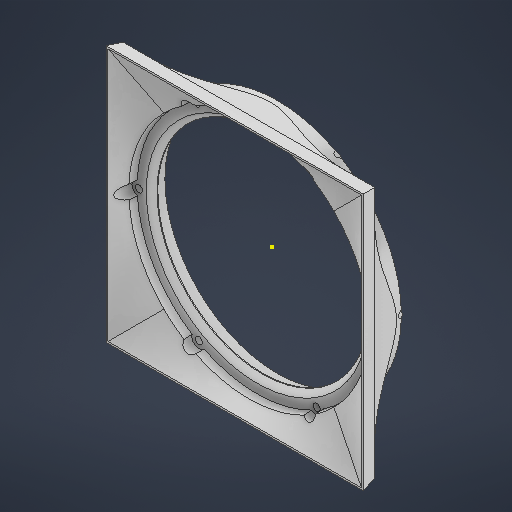
# Autodesk Inventor part: 供弹斜板
Saved by Autodesk Inventor 2025 (Build 290162000, 162)
## iProperties
Created: 2024-05-11
Part Number: 供弹斜板
Material: 常规
Document SubType Name: Modeling
Designer: HZD
Density: 1 g/cm^3
Appearance: 默认
Author: HZD
## iProperties of the stored document 供弹斜板_3D 打印.ipt
Created: 2024-07-10
Part Number: 供弹斜板_3D 打印
Material: 常规
Document SubType Name: Modeling
Designer: HZD
Density: 1 g/cm^3
Appearance: 默认
Author: HZD
Autodesk Inventor part; units mm, degrees
ref_plane "YZ Plane" through (0, 0, 0) normal (1, 0, 0) x (0, 1, 0)
ref_plane "XZ Plane" through (0, 0, 0) normal (0, 1, 0) x (-1, 0, 0)
ref_plane "工作平面1" through (0, 0, 20) normal (0, 0, 1) x (1, 0, 0)
sketch "草图30" plane through (-71.5017, -42.1486, 0) normal (0, 0, -1) x (-0.8614667, -0.5078141, 0)
  circle A0 centre (-83, 0) radius 64
  point P0 (-83, 0)
  dimension "d82" = 128
  constraints: 1 centre point, 1 coincident
  measures "d82" diameter of A0
sketch "草图19" plane through (0, 0, 3) normal (0, 0, 1) x (0.8718892, -0.4897032, 0)
  circle A0 centre (0, 0) radius 70.8 projected
  line L0 (-27.0916, -96.6485) -> (-93.2274, 21.1025)
  line L1 (98.0112, -26.2677) -> (-27.0916, -96.6485)
  line L2 (45.3823, -54.5376) -> (42.0698, -86.8145)
  line L3 (42.0698, -86.8145) -> (-27.0916, -96.6485)
  line L4 (-27.3263, -97.3539) -> (-18.3217, -65.2736) projected
  line L5 (-97.3643, 28.5723) -> (-27.1597, -96.6294)
  line L6 (-67.1338, -22.9554) -> (-81.1015, -52.2415)
  line L7 (-81.1015, -52.2415) -> (-27.1597, -96.6294)
  point P0 (34.788, -61.8361)
  point P1 (-61.8605, -34.7444)
  constraints: 14 end point, 4 symmetric about line, 4 other
sketch "草图21" plane through (-72.5, 72.5, 24) normal (0, 0, 1) x (1, 0, 0)
  circle A0 centre (72.5, -72.5) radius 70.95
  arc A1 (72.5499, -143.45) -> (1.55, -72.5) centre (72.5, -72.5) ccw projected
  line L0 (89.6905, -141.336) -> (42.9672, -149.9362)
  line L1 (42.9672, -149.9362) -> (-4.9362, -149.9362)
  line L2 (22.3308, -122.6692) -> (24.5608, -120.4392) projected
  line L3 (-4.9362, -149.9362) -> (22.3308, -122.6692)
  line L4 (3.664, -55.3095) -> (-4.9362, -102.0328)
  line L5 (-4.9362, -102.0328) -> (-4.9362, -149.9362)
  point P0 (80.9465, -142.9454)
  point P1 (2.0546, -64.0535)
  constraints: 10 end point, 2 symmetric about line, 1 centre point, 1 coincident, 1 horizontal, 1 point on circle
sketch "草图7" plane through (0, 0, 3) normal (0, 0, 1) x (1, 0, 0)
  circle A0 centre (-80.5933, -13.2719) radius 14.5326
  circle A1 centre (0, 0) radius 67.1463 projected
  constraints: 1 centre point, 1 tangent
sketch "草图2" plane through (0, 0, 0) normal (0, 0, 1) x (1, 0, 0)
  circle A0 centre (0, 0) radius 70
  dimension "d8" = 140
  constraints: 1 centre point, 1 coincident
  measures "d8" diameter of A0
sketch "草图3" plane through (0, 0, 20) normal (0, 0, 1) x (1, 0, 0)
  circle A0 centre (0, 0) radius 71
  dimension "d7" = 142
  constraints: 1 centre point, 1 coincident
  measures "d7" diameter of A0
loft "放样1" add profiles "草图2", "草图3"
shell "抽壳1" thickness 3 removed faces 1 at (12.047, 0, 20)
sketch "草图6" plane through (0, 0, 3) normal (0, 0, 1) x (1, 0, 0)
  circle A0 centre (0, 0) radius 63.4
  point P0 (0, 0)
  dimension "d97" = 126.8
  constraints: 1 centre point
  measures "d97" diameter of A0
extrude "拉伸2" cut sketch "草图6" against normal blind 38
sketch "草图9" plane through (0, 0, 20) normal (0, 0, 1) x (1, 0, 0)
  line L0 (71, 71) -> (-71, 71)
  line L1 (-71, 71) -> (-71, -71)
  line L2 (-71, -71) -> (71, -71)
  line L3 (71, -71) -> (71, 71)
  line L4 (71, 71) -> (-71, -71) construction
  line L5 (-71, 71) -> (71, -71) construction
  circle A0 centre (0, 0) radius 67.9963 projected
  dimension "d27" = 142
  dimension "d28" = 142
  constraints: 12 end point, 2 midpoint, 2 parallel, 1 horizontal, 1 perpendicular
  measures "d27" distance of L2.end L0.start
  measures "d28" distance of L0.start L0.end
extrude "拉伸4" add sketch "草图9" along normal blind 1
extrude "拉伸5" add sketch "草图9" against normal blind 4
fillet "圆角9" radius 19 1 edges at (-70.8, 0, 16)
ref_plane "工作平面2" through (0, 0, 24) normal (0, 0, 1) x (1, 0, 0)
sketch "草图12" plane through (0, 0, 16) normal (0, 0, -1) x (-1, 0, 0)
  line L0 (71, -71) -> (-71, -71) projected
  line L1 (71, 71) -> (-71, 71)
  line L2 (-71, 71) -> (-71, -71)
  line L3 (-71, -71) -> (71, -71)
  line L4 (71, -71) -> (71, 71)
  line L5 (71, 71) -> (-71, -71) construction
  line L6 (-71, 71) -> (71, -71) construction
  point P0 (0, 0)
  constraints: 12 end point, 2 midpoint, 2 parallel, 1 horizontal, 1 perpendicular
sketch "草图10" plane through (0, 0, 24) normal (0, 0, 1) x (1, 0, 0)
  line L0 (72.5, 72.5) -> (-72.5, 72.5)
  line L1 (-72.5, 72.5) -> (-72.5, -72.5)
  line L2 (-72.5, -72.5) -> (72.5, -72.5)
  line L3 (72.5, -72.5) -> (72.5, 72.5)
  line L4 (72.5, 72.5) -> (-72.5, -72.5) construction
  line L5 (-72.5, 72.5) -> (72.5, -72.5) construction
  point P0 (0, 0)
  dimension "d30" = 145
  dimension "d31" = 145
  constraints: 12 end point, 2 midpoint, 2 parallel, 1 horizontal, 1 perpendicular
  measures "d30" distance of L2.end L1.end
  measures "d31" distance of L0.end L1.end
loft "放样2" add profiles "草图12", "草图10"
sketch "草图13" plane through (-72.5, 72.5, 24) normal (0, 0, 1) x (1, 0, 0)
  line L0 (1, -1) -> (144, -1)
  line L1 (144, -1) -> (144, -144)
  line L2 (144, -144) -> (1, -144)
  line L3 (1, -144) -> (1, -1)
  line L4 (144, -1) -> (1, -1)
  line L5 (1, -1) -> (1, -144)
  line L6 (1, -144) -> (144, -144)
  line L7 (144, -144) -> (144, -1)
  line L8 (0, 0) -> (145, 0) projected
  line L9 (0, -145) -> (0, 0) projected
  line L10 (145, 0) -> (145, -145) projected
  line L11 (145, -145) -> (0, -145) projected
  point P0 (72.5, -72.5)
  dimension "d88" = 1
  dimension "d89" = 1
  dimension "d90" = 1
  dimension "d91" = 1
  constraints: 16 end point, 2 parallel, 1 horizontal, 1 perpendicular
  measures "d88" distance between parallel lines of L8 L0
  measures "d89" distance between parallel lines of L9 L3
  measures "d90" distance between parallel lines of L10 L1
  measures "d91" distance between parallel lines of L2 L11
sketch "草图15" plane through (0, 0, 16) normal (0, 0, -1) x (-1, 0, 0)
  circle A0 centre (0, 0) radius 67.7963 projected
  point P0 (0, 0)
loft "放样3" cut profiles "草图13", "草图15" contours L0 L1 L2 L3 / all
sketch "草图17" plane through (0, 0, 3) normal (0, 0, 1) x (1, 0, 0)
  circle A0 centre (33.7696, -57.2875) radius 2
  circle A1 centre (-32.7276, -57.8891) radius 2
  circle A2 centre (-66.4973, -0.6016) radius 2
  circle A3 centre (32.7276, 57.8891) radius 2
  circle A4 centre (66.4973, 0.6016) radius 1.65
  circle A5 centre (-33.7696, 57.2875) radius 1.65
  point P0 (0, 0)
  constraints: 6 centre point, 12 other
extrude "拉伸6" cut sketch "草图17" along normal mid plane 104
sketch "草图18" plane through (0, 0, 3) normal (0, 0, 1) x (0.8718892, -0.4897032, 0)
  point P0 (0, 0)
sketch "草图24" plane through (0, 0, 3) normal (0, 0, 1) x (0.8718892, -0.4897032, 0)
  circle A0 centre (0.1864, 66.4997) radius 2 projected
  circle A1 centre (0.1864, 66.4997) radius 4
  point P0 (0, 0)
  dimension "d63" = 8
  constraints: 1 centre point, 1 coincident
  measures "d63" diameter of A1
extrude "拉伸11" cut sketch "草图24" along normal blind 33.5 contours A0 | A1
pattern_circular "环形阵列1" count 6 over 360 about axis through (0, 0, -10) along (0, 0, 1) of "拉伸11"
sketch "草图27" plane through (0, 0, 3) normal (0, 0, 1) x (0.8614667, 0.5078141, 0)
  arc A0 (-58.8355, 37.0514) -> (-61.5194, 32.4983) centre (-57.5907, 33.25) ccw projected
  circle A1 centre (-57.5907, 33.25) radius 4
  circle A2 centre (0, 66.5) radius 1.65 projected
  circle A3 centre (0, 66.5) radius 4
  circle A4 centre (0, 0) radius 63.4 projected
  circle A5 centre (57.5907, 33.25) radius 2 projected
  circle A6 centre (57.5907, 33.25) radius 4.0042
  circle A7 centre (57.5907, -33.25) radius 1.65 projected
  circle A8 centre (57.5907, -33.25) radius 4
  circle A9 centre (0, -66.5) radius 2 projected
  circle A10 centre (0, -66.5) radius 4
  circle A11 centre (0, 0) radius 68.1203
  circle A12 centre (-57.5907, 33.25) radius 2 projected
  circle A13 centre (-57.5907, -33.25) radius 2 projected
  circle A14 centre (-57.5907, -33.25) radius 4.0197
  point P0 (0, 0)
  point P1 (60.759, 30.8014)
  point P2 (57.0543, 37.2181)
  point P3 (3.7, 68.0198)
  point P4 (-3.7, 68.0198)
  point P5 (-57.0568, 37.2142)
  point P6 (-58.8355, 37.0514)
  point P7 (-61.5194, 32.4983)
  point P8 (-60.7569, 30.8056)
  point P9 (-60.7667, -30.7862)
  point P10 (-57.0449, -37.2324)
  point P11 (-3.7, -68.0198)
  point P12 (3.7, -68.0198)
  point P13 (57.0568, -37.2142)
  point P14 (60.7569, -30.8056)
  point P15 (58.8357, -34.3328)
  point P16 (59.1509, -33.7868)
  point P17 (2.4678, 63.352)
  point P18 (56.0983, -29.5388)
  point P19 (53.6305, -33.8131)
  point P20 (-56.0983, 29.5388)
  point P21 (-53.6305, 33.8131)
  point P22 (-2.4678, 63.352)
  point P23 (-59.5783, 33.0274)
  point P24 (-58.3917, 35.0826)
  point P25 (-58.3917, -35.0826)
  point P26 (-59.5783, -33.0274)
  point P27 (-1.1866, -68.11)
  point P28 (1.1866, -68.11)
  point P29 (-0.3153, 68.1196)
  point P30 (0.3153, 68.1196)
  point P31 (58.3917, 35.0826)
  point P32 (59.5783, 33.0274)
  constraints: 7 coincident, 6 centre point, 2 horizontal alignment, 1 concentric, 4 other
extrude "拉伸15" add sketch "草图27" along normal blind 8.5 contours A1 A11 A12 A0 | A11 A3 A4 A1 | A1 A4 A11 A12 | A1 A4 A14 A11 | A11 A2 A3 A4 | A3 A11 A2 | A14 A4 A11 A13 | A11 A13 A14 | A11 A6 A4 A3 | A14 A4 A10 A11 | A11 A5 A6 A4 | A6 A11 A5 | A11 A9 A10 | A10 A4 A11 A9 | A10 A4 A8 A11 | A6 A11 A8 A4 | A11 A7 A8 | A8 A4 A11 A7
extrude "拉伸16" add sketch "草图27" against normal up to surface (3 mm away) contours A1 A11 A12 A0 | A3 A11 A2 | A11 A13 A14 | A6 A11 A5 | A11 A9 A10 | A11 A7 A8
sketch "草图29" plane through (0, 0, 11.5) normal (0, 0, 1) x (0.8614667, 0.5078141, 0)
  circle A0 centre (0, 0) radius 63.4 projected
  circle A1 centre (0, 0) radius 59.4
  point P0 (0, 0)
  dimension "d79" = 4
  constraints: 1 centre point
  measures "d79" radial gap between concentric circles of A0 A1
extrude "拉伸17" add sketch "草图29" against normal blind 3.5
chamfer "倒角2" distance 3 angle 45 1 edges at (-51.1711, -30.1642, 11.5)
